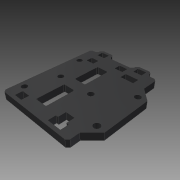
# Autodesk Inventor part: x_motor_top
Saved by Autodesk Inventor 2014 (Build 180170000, 170)
## iProperties
Created: 2013-12-01
Part Number: x_motor_top
Material: Generic
Document SubType Name: Modeling
Designer: buben
Density: 1 g/cm^3
Appearance: Anodized - Dark Gray
Author: buben
Subject: Laser Cutted
Autodesk Inventor part; units mm, degrees
ref_plane "YZ Plane" through (0, 0, 0) normal (1, 0, 0) x (0, 1, 0)
ref_plane "XZ Plane" through (0, 0, 0) normal (0, 1, 0) x (-1, 0, 0)
ref_plane "XY Plane" through (0, 0, 0) normal (0, 0, 1) x (1, 0, 0)
sketch "Sketch1" plane through (0, 0, 0) normal (0, 0, 1) x (1, 0, 0)
  line L0 (0, 0) -> (68, 0)
  line L1 (68, 87.5) -> (0, 87.5)
  line L2 (0, 87.5) -> (0, 0)
  line L3 (68, 71.5) -> (78, 61.5)
  line L4 (78, 61.5) -> (78, 19.5)
  line L5 (78, 19.5) -> (68, 9.5)
  line L6 (68, 0) -> (68, 9.5)
  line L7 (68, 71.5) -> (68, 87.5)
  line L8 (35, 84.5) -> (43, 84.5)
  line L9 (43, 84.5) -> (43, 78)
  line L10 (43, 78) -> (35, 78)
  line L11 (35, 78) -> (35, 84.5)
  line L12 (10, 78) -> (18, 78)
  line L13 (18, 78) -> (18, 71.5)
  line L14 (18, 71.5) -> (10, 71.5)
  line L15 (10, 71.5) -> (10, 78)
  line L16 (10, 9.5) -> (18, 9.5)
  line L17 (18, 9.5) -> (18, 3)
  line L18 (18, 3) -> (10, 3)
  line L19 (10, 3) -> (10, 9.5)
  line L20 (25, 70.5) -> (34, 70.5)
  line L21 (35, 69.5) -> (35, 46.5)
  line L22 (34, 45.5) -> (25, 45.5)
  line L23 (24, 46.5) -> (24, 69.5)
  line L24 (25, 35.5) -> (34, 35.5)
  line L25 (35, 34.5) -> (35, 11.5)
  line L26 (34, 10.5) -> (25, 10.5)
  line L27 (24, 11.5) -> (24, 34.5)
  arc A0 (25, 70.5) -> (24, 69.5) centre (25, 69.5) ccw
  arc A1 (35, 69.5) -> (34, 70.5) centre (34, 69.5) ccw
  arc A2 (34, 45.5) -> (35, 46.5) centre (34, 46.5) ccw
  arc A3 (24, 46.5) -> (25, 45.5) centre (25, 46.5) ccw
  arc A4 (25, 35.5) -> (24, 34.5) centre (25, 34.5) ccw
  arc A5 (24, 11.5) -> (25, 10.5) centre (25, 11.5) ccw
  arc A6 (34, 10.5) -> (35, 11.5) centre (34, 11.5) ccw
  arc A7 (35, 34.5) -> (34, 35.5) centre (34, 34.5) ccw
  line L28 (29.5, 70.5) -> (29.5, 10.5) construction
  circle A8 centre (71, 60.5) radius 2.75
  circle A9 centre (71, 20.5) radius 2.75
  line L29 (46.5, 3) -> (58.5, 3)
  line L30 (58.5, 3) -> (58.5, 9.5)
  line L31 (58.5, 9.5) -> (46.5, 9.5)
  line L32 (46.5, 9.5) -> (46.5, 3)
  circle A10 centre (6, 13.5) radius 5 construction
  circle A11 centre (6, 13.5) radius 2.75
  circle A12 centre (6, 67.5) radius 5 construction
  circle A13 centre (6, 67.5) radius 2.75
  line L33 (46.5, 78) -> (58.5, 78)
  line L34 (58.5, 78) -> (58.5, 71.5)
  line L35 (58.5, 71.5) -> (46.5, 71.5)
  line L36 (46.5, 71.5) -> (46.5, 78)
  line L37 (21, 84.5) -> (29, 84.5)
  line L38 (29, 84.5) -> (29, 78)
  line L39 (29, 78) -> (21, 78)
  line L40 (21, 78) -> (21, 84.5)
  circle A14 centre (71, 60.5) radius 5 construction
  circle A15 centre (71, 20.5) radius 5 construction
  circle A16 centre (14, 40.5) radius 5 construction
  circle A17 centre (46, 40.5) radius 5 construction
  circle A18 centre (46, 40.5) radius 2.75
  circle A19 centre (14, 40.5) radius 2.75
  line L41 (50, 87.5) -> (50, 0) construction
  line L42 (55, 87.5) -> (55, 0) construction
  line L43 (52.5, 87.5) -> (52.5, 0) construction
  line L44 (72, 13.5) -> (0, 13.5) construction
  line L45 (72, 67.5) -> (0, 67.5) construction
  point P0 (78, 40.5)
  point P1 (52.5, 3)
  dimension "d1" = 45
  dimension "d2" = 10
  dimension "d3" = 6.5
  dimension "d4" = 6.5
  dimension "d5" = 8
  dimension "d6" = 8
  dimension "d7" = 3
  dimension "d8" = 6.5
  dimension "d9" = 3
  dimension "d12" = 1
  dimension "d13" = 11
  dimension "d14" = 25
  dimension "d15" = 25
  dimension "d16" = 1
  dimension "d17" = 1
  dimension "d18" = 38.5
  dimension "d19" = 5.5
  dimension "d20" = 5.5
  dimension "d21" = 7
  dimension "d24" = 12
  dimension "d25" = 11
  dimension "d26" = 11
  dimension "d27" = 10
  dimension "d28" = 5.5
  dimension "d29" = 5.5
  dimension "d30" = 10
  dimension "d32" = 4
  dimension "d33" = 4
  dimension "d34" = 4
  dimension "d35" = 6
  dimension "d36" = 68
  dimension "d39" = 8
  dimension "d40" = 3
  dimension "d41" = 10
  dimension "d42" = 10
  dimension "d43" = 4
  dimension "d44" = 10
  dimension "d45" = 5.5
  dimension "d46" = 10
  dimension "d47" = 5.5
  dimension "d49" = 14
  dimension "d50" = 32
  dimension "d51" = 5
  dimension "d52" = 2.5
  dimension "d53" = 15.5
  dimension "d92" = 4
  dimension "d93" = 4
  dimension "d94" = 54
  dimension "d95" = 6
  constraints: 92 end point, 22 parallel, 20 centre point, 16 point on circle, 16 tangent, 15 perpendicular, 13 collinear, 10 point on line, 9 horizontal, 7 equal radius, 6 coincident, 4 horizontal alignment, 4 midpoint, 2 vertical alignment
  measures "d1" angle of L7 L3
  measures "d2" distance between parallel lines of L7 L4
  measures "d3" distance of L14.end L12.start
  measures "d4" distance of L10.end L8.start
  measures "d5" distance of L12.start L12.end
  measures "d6" distance of L8.start L8.end
  measures "d7" distance between parallel lines of L1 L8
  measures "d8" distance of L18.end L16.start
  measures "d9" distance between parallel lines of L0 L18
  measures "d12" radius of A0
  measures "d13" distance between parallel lines of L21 L23
  measures "d14" distance between parallel lines of L20 L22
  measures "d15" distance between parallel lines of L26 L24
  measures "d16" distance between parallel lines of L20 L14
  measures "d17" distance between parallel lines of L26 L16
  measures "d18" distance between parallel lines of L7 L28
  measures "d19" diameter of A8
  measures "d20" diameter of A9
  measures "d21" distance from line of L4 A9.centre
  measures "d24" distance of L30.end L31.end
  measures "d25" vertical distance of A9.centre L5.end
  measures "d26" vertical distance of L3.start A8.centre
  measures "d27" diameter of A12
  measures "d28" diameter of A13
  measures "d29" diameter of A11
  measures "d30" diameter of A10
  measures "d32" distance from line of L14 A12.centre
  measures "d33" distance from line of L19 A10.centre
  measures "d34" distance from line of L16 A10.centre
  measures "d35" distance from line of L2 A12.centre
  measures "d36" distance of L0.start L0.end
  measures "d39" distance of L38.end L39.end
  measures "d40" distance between parallel lines of L13 L40
  measures "d41" diameter of A14
  measures "d42" diameter of A15
  measures "d43" distance from line of L15 A12.centre
  measures "d44" diameter of A16
  measures "d45" diameter of A19
  measures "d46" diameter of A17
  measures "d47" diameter of A18
  measures "d49" distance from line of L2 A16.centre
  measures "d50" distance from line of L4 A17.centre
  measures "d51" distance between parallel lines of L41 L42
  measures "d52" distance between parallel lines of L41 L43
  measures "d53" distance between parallel lines of L6 L43
  measures "d92" distance between parallel lines of L44 L16
  measures "d93" distance between parallel lines of L14 L45
  measures "d94" distance between parallel lines of L44 L45
  measures "d95" distance between parallel lines of L11 L38
extrude "Extrusion1" add sketch "Sketch1" along normal blind 6.5
chamfer "Chamfer1" distance 2 angle 45 4 edges at (0, 0, 3.25) (68, 0, 3.25) (68, 87.5, 3.25) (0, 87.5, 3.25)
sketch "Sketch2" plane through (0, 0, 6.5) normal (0, 0, 1) x (1, 0, 0)
  line L0 (46.5, 9.5) -> (58.5, 9.5) projected
  line L1 (68, 2) -> (68, 9.5) projected
  line L2 (48.5, 16) -> (56.5, 16)
  line L3 (56.5, 16) -> (56.5, 9.5)
  line L4 (56.5, 9.5) -> (48.5, 9.5)
  line L5 (48.5, 9.5) -> (48.5, 16)
  point P0 (0, 0)
  dimension "d59" = 6.5
  dimension "d60" = 8
  dimension "d63" = 11.5
  constraints: 8 end point, 2 parallel, 1 collinear, 1 horizontal, 1 perpendicular
  measures "d59" distance of L4.end L2.start
  measures "d60" distance of L2.start L2.end
  measures "d63" distance between parallel lines of L1 L3
extrude "Extrusion2" cut sketch "Sketch2" against normal through all
sketch "Sketch3" plane through (0, 0, 6.5) normal (0, 0, 1) x (1, 0, 0)
  line L0 (29, 84.5) -> (29, 78) projected
  line L1 (29, 78) -> (21, 78) projected
  line L2 (21, 78) -> (21, 84.5) projected
  line L3 (21, 84.5) -> (29, 84.5) projected
  point P0 (0, 0)
extrude "Extrusion3" add sketch "Sketch3" against normal blind 6.5
sketch "Sketch6" plane through (0, 0, 6.5) normal (0, 0, 1) x (1, 0, 0)
  line L0 (18, 78) -> (18, 71.5) projected
  line L1 (10, 71.5) -> (10, 78) projected
  line L2 (66, 87.5) -> (2, 87.5) projected
  line L3 (7, 87.5) -> (21, 87.5)
  line L4 (21, 87.5) -> (21, 93.5)
  line L5 (21, 93.5) -> (7, 93.5)
  line L6 (7, 93.5) -> (7, 87.5)
  line L7 (45.5, 87.5) -> (59.5, 87.5)
  line L8 (59.5, 87.5) -> (59.5, 93.5)
  line L9 (59.5, 93.5) -> (45.5, 93.5)
  line L10 (45.5, 93.5) -> (45.5, 87.5)
  line L11 (46.5, 78) -> (58.5, 78) projected
  point P0 (0, 0)
  point P1 (52.5, 93.5)
  point P2 (52.5, 78)
  dimension "d80" = 3
  dimension "d81" = 3
  dimension "d84" = 6
  constraints: 16 end point, 4 parallel, 2 collinear, 2 horizontal, 2 midpoint, 2 perpendicular, 2 point on line, 1 vertical alignment
  measures "d80" distance between parallel lines of L1 L6
  measures "d81" distance between parallel lines of L4 L0
  measures "d84" distance of L5.end L3.start
extrude "Extrusion6" add sketch "Sketch6" against normal blind 6.5
sketch "Sketch7" plane through (0, 0, 6.5) normal (0, 0, 1) x (1, 0, 0)
  line L0 (18, 78) -> (18, 71.5) projected
  line L1 (10, 71.5) -> (10, 78) projected
  line L2 (43, 84.5) -> (43, 78) projected
  line L3 (35, 78) -> (35, 84.5) projected
  line L4 (35, 84.5) -> (43, 84.5) projected
  line L5 (10, 91) -> (18, 91)
  line L6 (18, 91) -> (18, 84.5)
  line L7 (18, 84.5) -> (10, 84.5)
  line L8 (10, 84.5) -> (10, 91)
  line L9 (48.5, 91) -> (56.5, 91)
  line L10 (56.5, 91) -> (56.5, 84.5)
  line L11 (56.5, 84.5) -> (48.5, 84.5)
  line L12 (48.5, 84.5) -> (48.5, 91)
  line L13 (59.5, 93.5) -> (45.5, 93.5) projected
  point P0 (0, 0)
  point P1 (52.5, 91)
  point P2 (52.5, 93.5)
  constraints: 16 end point, 4 collinear, 4 parallel, 3 equal length, 2 horizontal, 2 midpoint, 2 perpendicular, 1 vertical alignment
extrude "Extrusion7" cut sketch "Sketch7" against normal blind 6.5
chamfer "Chamfer3" distance 2 angle 45 8 edges at (7, 87.5, 3.25) (7, 93.5, 3.25) (21, 93.5, 3.25) (21, 87.5, 3.25) (45.5, 87.5, 3.25) (45.5, 93.5, 3.25) (59.5, 93.5, 3.25) (59.5, 87.5, 3.25)
body "Solid1"
